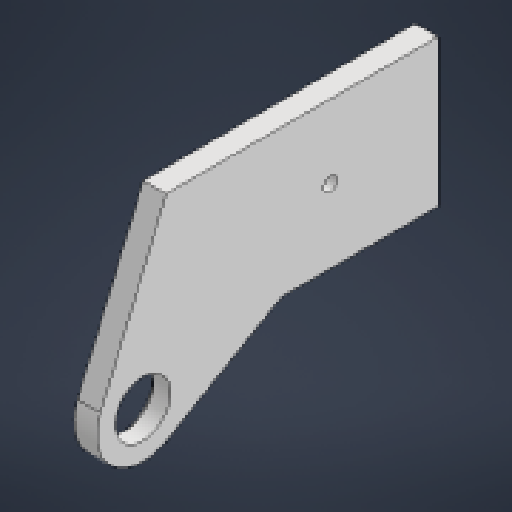
# Autodesk Inventor part: Gear_Frame
Saved by Autodesk Inventor 2024.2 (Build 282272000, 272)
## iProperties
Created: 2023-12-27
Part Number: Gear_Frame
Material: 一般
Document SubType Name: Modeling
Designer: Hanaoka
Density: 1 g/cm^3
Appearance: 既定
Author: Hanaoka
Autodesk Inventor part; units mm, degrees
ref_plane "YZ Plane" through (0, 0, 0) normal (1, 0, 0) x (0, 1, 0)
ref_plane "XZ Plane" through (0, 0, 0) normal (0, 1, 0) x (-1, 0, 0)
ref_plane "XY Plane" through (0, 0, 0) normal (0, 0, 1) x (1, 0, 0)
sketch "スケッチ1" plane through (0, 0, 0) normal (1, 0, 0) x (0, 1, 0)
  circle A0 centre (0, 0) radius 5 construction
  circle A1 centre (0, 0) radius 3.6
  arc A2 (1.9342, 4.6107) -> (-4.3208, -2.5162) centre (0, 0) ccw
  line L0 (-4.3208, -2.5162) -> (3, -15.0874)
  line L1 (3, -15.0874) -> (3, -32.1321)
  line L2 (3, -32.1321) -> (19, -32.1321)
  line L3 (19, -32.1321) -> (19, -2.5484)
  line L4 (19, -2.5484) -> (1.9342, 4.6107)
  circle A3 centre (0, 0) radius 3
  circle A4 centre (11, -20.4215) radius 0.75
  circle A5 centre (11, -20.4215) radius 5 construction
  circle A6 centre (16, -20.4215) radius 1 construction
  line L5 (16, -20.4215) -> (6, -20.4215) construction
  circle A7 centre (6, -20.4215) radius 1 construction
  circle A8 centre (11, -20.4215) radius 8 construction
  dimension "d1" = 10
  dimension "d0" = 7.2
  dimension "d4" = 6
  dimension "d7" = 1.5
  dimension "d8" = 10
  dimension "d9" = 2
  dimension "d11" = 16
  constraints: 12 end point, 8 centre point, 7 coincident, 4 point on circle, 2 horizontal, 2 tangent, 2 vertical, 1 equal radius, 1 midpoint, 1 point on line, 6 other
  measures "d0" diameter of A1
  measures "d4" diameter of A3
  measures "d7" diameter of A4
  measures "d8" diameter of A5
  measures "d9" diameter of A6
  measures "d11" diameter of A8
extrude "押し出し1" add sketch "スケッチ1" along normal blind 2.5 contours A1 | L4 L3 L2 L1 L0 A2
extrude "押し出し2" cut sketch "スケッチ1" along normal blind 0.6 contours A1 | A3
